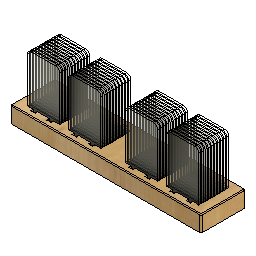
LED-Nixie-Clock (Autodesk Fusion 360 design; units mm, degrees)
Autodesk Fusion 360 part; units mm, degrees
note: some values were not read from the file. Chosen so that the rebuilt part matches the saved one: which face or edge a step refers to; how an offset face is resized. Set by a fixed rule: which sketch regions a step uses.
sketch "Skizze1" plane through (0, 0, 0) normal (0, 0, 1) x (1, 0, 0) in component "Digit"
  line L0 (-15, 60) -> (15, 60)
  line L1 (20, 55) -> (20, 0)
  line L2 (-20, 55) -> (-20, 0)
  line L3 (-20, 0) -> (-20, -10)
  line L4 (-20, -10) -> (20, -10)
  line L5 (20, -10) -> (20, 0)
  line L6 (-20, 0) -> (20, 0)
  arc A0 (-15, 60) -> (-20, 55) centre (-15, 55) ccw
  arc A1 (20, 55) -> (15, 60) centre (15, 55) ccw
  circle A2 centre (-10, -4.35) radius 1.65
  circle A3 centre (10, -4.35) radius 1.65
  line L7 (-20, -6) -> (20, -6) construction
  dimension "d8" = 10
  dimension "d9" = 5
  dimension "d10" = 5
  dimension "d11" = 60
  dimension "d12" = 40
  dimension "d96" = 3.3
  dimension "d97" = 3.3
  dimension "d124" = 6
  measures "d8" distance of origin
  measures "d9" radius of A0
  measures "d10" radius of A1
  measures "d11" distance of L0 L6
  measures "d12" distance of L1 L2
  measures "d96" diameter of A2
  measures "d97" diameter of A3
  measures "d124" distance of L6 L7
extrude "Extrusion1" add sketch "Skizze1" along normal blind 2.5 makes body 1 in component "Digit"
sketch "Skizze1 (2)" plane through (0, 0, 2.5) normal (0, 0, 1) x (-1, 0, 0) in component "Digit Spacer"
  circle A0 centre (10, 4.35) radius 1.65
  circle A1 centre (-10, 4.35) radius 1.65
  arc A2 (15, -60) -> (20, -55) centre (15, -55) ccw
  line L0 (20, -55) -> (20, 0)
  line L1 (20, 0) -> (20, 10)
  line L2 (20, 10) -> (-20, 10)
  line L3 (-20, 10) -> (-20, -55)
  arc A3 (-20, -55) -> (-15, -60) centre (-15, -55) ccw
  line L4 (-15, -60) -> (15, -60)
  circle A4 centre (10, 4.35) radius 1.65
  circle A5 centre (-10, 4.35) radius 1.65
  line L5 (20, 0) -> (-20, 0)
  line L6 (-20, 10) -> (-20, 0)
  line L7 (20, 10) -> (-20, 10)
  line L8 (20, 0) -> (20, 10)
extrude "Extrusion1'" add sketch "Skizze1 (2)" along normal blind 1.31 separate body contours L1 L2 L3 L5 L6 L7 L8 makes body 2 in component "Digit Spacer"
pattern_linear "R-Anordnung3" [suppressed]
pattern_linear "R-Anordnung6" [suppressed]
sketch "Skizze1 (3)" plane through (0, 0, 0) normal (0, 0, 1) x (1, 0, 0) in component "Digit Screw"
  circle A0 centre (0, 0) radius 1.5
  circle A1 centre (0, 0) radius 2.75
  line L0 (1.4382, 0.1218) -> (0.6136, 1.3064)
  line L1 (0.6136, 1.3064) -> (-0.8246, 1.1846)
  line L2 (-0.8246, 1.1846) -> (-1.4382, -0.1218)
  line L3 (-1.4382, -0.1218) -> (-0.6136, -1.3064)
  line L4 (-0.6136, -1.3064) -> (0.8246, -1.1846)
  line L5 (0.8246, -1.1846) -> (1.4382, 0.1218)
  line L6 (1.4064, 2.847) -> (-1.7623, 2.6415)
  line L7 (-1.7623, 2.6415) -> (-3.1688, -0.2055)
  line L8 (-3.1688, -0.2055) -> (-1.4064, -2.847)
  line L9 (-1.4064, -2.847) -> (1.7623, -2.6415)
  line L10 (1.7623, -2.6415) -> (3.1688, 0.2055)
  line L11 (3.1688, 0.2055) -> (1.4064, 2.847)
  dimension "d107" = 3
  dimension "d108" = 5.5
  dimension "d109" = 1.25
  dimension "d116" = 2.75
  measures "d107" diameter of A0
  measures "d108" diameter of A1
  measures "d109" distance of A0.centre L5
  measures "d116" distance of A0.centre L11
extrude "Extrusion1''" add sketch "Skizze1 (3)" against normal blind 3 separate body contours A0 | A1 makes body 3 in component "Digit Screw"
extrude "Extrusion2" add sketch "Skizze1 (3)" along normal blind 40 contours A0 | L0 L1 L2 L3 L4 L5 bodies 3 in component "Digit Screw"
thread "Gewinde1" "ISO Metric profile 3.0 M3x0.5 6g" major diameter 2.927 minor diameter 2.3555 pitch 0.5 angle 60 resizes the face on face at (1.4981, -0.0748, 26.6667) on bodies 3 in component "Digit Screw"
extrude "Extrusion3" add sketch "Skizze1 (3)" along normal blind 2.4 from surface at 36.79 separate body contours A1 | A1 L10 L11 | A1 L6 L11 | A1 L9 L10 | A1 L6 L7 | A1 L8 L9 | A1 L7 L8 makes body 4 in component "Digit Screw"
pattern_linear "R-Anordnung4" [suppressed]
pattern_linear "R-Anordnung5" [suppressed]
sketch "Skizze1 (4)" plane through (0, 0, 0) normal (0, 0, 1) x (1, 0, 0) in component "Base"
  line L0 (-20, 0) -> (-20, -36.79)
  line L1 (191.45, -36.79) -> (191.45, 0)
  line L2 (-31.775, 9.105) -> (203.225, 9.105)
  line L3 (203.225, 9.105) -> (203.225, -45.895)
  line L4 (203.225, -45.895) -> (-31.775, -45.895)
  line L5 (-31.775, -45.895) -> (-31.775, 9.105)
  line L6 (-12.75, -39.79) -> (-7.25, -39.79)
  line L7 (7.25, -39.79) -> (12.75, -39.79)
  line L8 (38.05, -39.79) -> (43.55, -39.79)
  line L9 (58.05, -39.79) -> (63.55, -39.79)
  line L10 (107.9, -39.79) -> (113.4, -39.79)
  line L11 (127.9, -39.79) -> (133.4, -39.79)
  line L12 (158.7, -39.79) -> (164.2, -39.79)
  line L13 (178.7, -39.79) -> (184.2, -39.79)
  line L14 (-12.75, -39.79) -> (-12.75, -36.79)
  line L15 (-7.25, -39.79) -> (-7.25, -36.79)
  line L16 (7.25, -39.79) -> (7.25, -36.79)
  line L17 (12.75, -36.79) -> (12.75, -39.79)
  line L18 (38.05, -36.79) -> (38.05, -39.79)
  line L19 (43.55, -39.79) -> (43.55, -36.79)
  line L20 (58.05, -39.79) -> (58.05, -36.79)
  line L21 (63.55, -36.79) -> (63.55, -39.79)
  line L22 (107.9, -36.79) -> (107.9, -39.79)
  line L23 (113.4, -39.79) -> (113.4, -36.79)
  line L24 (127.9, -36.79) -> (127.9, -39.79)
  line L25 (133.4, -39.79) -> (133.4, -36.79)
  line L26 (158.7, -36.79) -> (158.7, -39.79)
  line L27 (164.2, -36.79) -> (164.2, -39.79)
  line L28 (178.7, -36.79) -> (178.7, -39.79)
  line L29 (184.2, -39.79) -> (184.2, -36.79)
  line L30 (20, 0) -> (20, -36.79)
  line L31 (-20, 0) -> (20, 0)
  line L32 (30.8, 0) -> (30.8, -36.79)
  line L33 (70.8, -36.79) -> (70.8, 0)
  line L34 (70.8, 0) -> (30.8, 0)
  line L35 (100.65, -36.79) -> (100.65, 0)
  line L36 (100.65, 0) -> (140.65, 0)
  line L37 (140.65, 0) -> (140.65, -36.79)
  line L38 (151.45, -36.79) -> (151.45, 0)
  line L39 (151.45, 0) -> (191.45, 0)
  line L40 (-21.775, 3.605) -> (193.225, 3.605)
  line L41 (193.225, 3.605) -> (193.225, -40.395)
  line L42 (193.225, -40.395) -> (-21.775, -40.395)
  line L43 (-21.775, -40.395) -> (-21.775, 3.605)
  line L44 (85.725, 0) -> (85.725, 3.605) construction
  line L45 (70.8, 0) -> (100.65, 0) construction
  line L46 (85.725, 3.605) -> (85.725, 9.105) construction
  line L47 (-20, -18.395) -> (-21.775, -18.395) construction
  line L48 (-21.775, -18.395) -> (-31.775, -18.395) construction
  line L49 (-20, -18.395) -> (20, -18.395) construction
  line L50 (-12.75, 3) -> (-12.75, 0)
  line L51 (-12.75, 3) -> (-7.25, 3)
  line L52 (-7.25, 3) -> (-7.25, 0)
  line L53 (7.25, 3) -> (7.25, 0)
  line L54 (7.25, 3) -> (12.75, 3)
  line L55 (12.75, 0) -> (12.75, 3)
  line L56 (30.8, -18.395) -> (70.8, -18.395) construction
  line L57 (100.65, -18.395) -> (140.65, -18.395) construction
  line L58 (151.45, -18.395) -> (191.45, -18.395) construction
  line L59 (38.05, 0) -> (38.05, 3)
  line L60 (38.05, 3) -> (43.55, 3)
  line L61 (43.55, 3) -> (43.55, 0)
  line L62 (58.05, 3) -> (58.05, 0)
  line L63 (58.05, 3) -> (63.55, 3)
  line L64 (63.55, 0) -> (63.55, 3)
  line L65 (107.9, 0) -> (107.9, 3)
  line L66 (107.9, 3) -> (113.4, 3)
  line L67 (113.4, 3) -> (113.4, 0)
  line L68 (127.9, 0) -> (127.9, 3)
  line L69 (127.9, 3) -> (133.4, 3)
  line L70 (133.4, 3) -> (133.4, 0)
  line L71 (158.7, 0) -> (158.7, 3)
  line L72 (158.7, 3) -> (164.2, 3)
  line L73 (164.2, 0) -> (164.2, 3)
  line L74 (178.7, 0) -> (178.7, 3)
  line L75 (178.7, 3) -> (184.2, 3)
  line L76 (184.2, 3) -> (184.2, 0)
  line L77 (-20, -36.79) -> (20, -36.79)
  line L78 (30.8, -36.79) -> (70.8, -36.79)
  line L79 (100.65, -36.79) -> (140.65, -36.79)
  line L80 (151.45, -36.79) -> (191.45, -36.79)
  dimension "d122" = 55
  dimension "d123" = 235
  dimension "d147" = 215
  dimension "d148" = 44
  measures "d122" distance of origin
  measures "d148" distance of origin
extrude "Extrusion6" add sketch "Skizze1 (4)" against normal blind 20 separate body contours L0 L30 L31 L77 | L31 L50 L51 L52 | L6 L14 L15 L77 | L31 L53 L54 L55 | L7 L16 L17 L77 | L1 L38 L39 L80 | L13 L28 L29 L80 | L39 L74 L75 L76 | L12 L26 L27 L80 | L39 L71 L72 L73 | L2 L3 L4 L5 | L8 L18 L19 L78 | L32 L33 L34 L78 | L9 L20 L21 L78 | L34 L59 L60 L61 | L34 L62 L63 L64 | L10 L22 L23 L79 | L35 L36 L37 L79 | L11 L24 L25 L79 | L36 L65 L66 L67 | L36 L68 L69 L70 | L40 L41 L42 L43 makes body 5 in component "Base"
extrude "Extrusion9" cut sketch "Skizze1 (4)" against normal blind 10 contours L0 L30 L31 L77 | L1 L38 L39 L80 | L32 L33 L34 L78 | L35 L36 L37 L79 bodies 5 in component "Base"
extrude "Extrusion10" cut sketch "Skizze1 (4)" against normal blind 7.5 contours L31 L50 L51 L52 | L6 L14 L15 L77 | L31 L53 L54 L55 | L7 L16 L17 L77 | L13 L28 L29 L80 | L39 L74 L75 L76 | L12 L26 L27 L80 | L39 L71 L72 L73 | L8 L18 L19 L78 | L9 L20 L21 L78 | L34 L59 L60 L61 | L34 L62 L63 L64 | L10 L22 L23 L79 | L11 L24 L25 L79 | L36 L65 L66 L67 | L36 L68 L69 L70 bodies 5 in component "Base"
extrude "Extrusion11" cut sketch "Skizze1 (4)" against normal blind 10 from surface at -10 contours L0 L30 L31 L77 | L31 L50 L51 L52 | L6 L14 L15 L77 | L31 L53 L54 L55 | L7 L16 L17 L77 | L1 L38 L39 L80 | L13 L28 L29 L80 | L39 L74 L75 L76 | L12 L26 L27 L80 | L39 L71 L72 L73 | L8 L18 L19 L78 | L32 L33 L34 L78 | L9 L20 L21 L78 | L34 L59 L60 L61 | L34 L62 L63 L64 | L10 L22 L23 L79 | L35 L36 L37 L79 | L11 L24 L25 L79 | L36 L65 L66 L67 | L36 L68 L69 L70 | L40 L41 L42 L43 bodies 5 in component "Base"
hole "Bohrung2" at (76.3217, 9.105, -19.9759) direction (0, -1, 0) diameter 10 depth 10 tip angle 180 bodies 5 in component "Base"
fillet "Abrundung2" radius 2 4 edges at (-31.775, -45.895, -10) (-31.775, 9.105, -10) (203.225, 9.105, -10) (203.225, -45.895, -10) on bodies 5 in component "Base"
chamfer "Fase2" distance 1 angle 45 8 edges at (-31.775, -18.395, 0) (-31.1892, 8.5192, 0) (85.725, 9.105, 0) (202.6392, 8.5192, 0) (203.225, -18.395, 0) (202.6392, -45.3092, 0) (85.725, -45.895, 0) (-31.1892, -45.3092, 0) on bodies 5 in component "Base"
sketch "Skizze1 (5)" plane through (0, 0, 0) normal (0, 0, 1) x (1, 0, 0) in component "PCB"
  line L0 (0, 0) -> (214.63, 0)
  line L1 (214.63, 0) -> (214.63, -43.18)
  line L2 (214.63, -43.18) -> (0, -43.18)
  line L3 (0, -43.18) -> (0, 0)
  line L4 (107.315, 0) -> (107.315, -43.18) construction
  line L5 (0, -3.17) -> (214.63, -3.17) construction
  line L6 (0, -40.01) -> (214.63, -40.01) construction
  circle A0 centre (107.315, -3.17) radius 1.65
  circle A1 centre (107.315, -40.01) radius 1.65
  line L7 (46.985, 0) -> (46.985, -43.18) construction
  line L8 (167.645, 0) -> (167.645, -43.18) construction
  circle A2 centre (46.985, -3.17) radius 1.65
  circle A3 centre (46.985, -40.01) radius 1.65
  circle A4 centre (167.645, -3.17) radius 1.65
  circle A5 centre (167.645, -40.01) radius 1.65
  dimension "d154" = 43.18
  dimension "d155" = 214.63
  dimension "d156" = 3.17
  dimension "d157" = 3.17
  dimension "d158" = 3.3
  dimension "d159" = 3.3
  dimension "d160" = 60.33
  dimension "d161" = 60.33
  dimension "d162" = 3.3
  dimension "d163" = 3.3
  dimension "d164" = 3.3
  dimension "d165" = 3.3
  measures "d154" distance of L0.start
  measures "d155" distance of L0.start
  measures "d156" distance of L0 L5
  measures "d157" distance of L2 L6
  measures "d158" diameter of A0
  measures "d159" diameter of A1
  measures "d160" distance of L4 L7
  measures "d161" distance of L4 L8
  measures "d162" diameter of A2
  measures "d163" diameter of A3
  measures "d164" diameter of A4
  measures "d165" diameter of A5
extrude "Extrusion1'''" add sketch "Skizze1 (5)" along normal blind 1.6 separate body makes body 6 in component "PCB"
component "Digit" placed x (1, 0, 0) y (0, 0, 1) z (0, -1, 0) at (0, 0, 0)
component "Digit Spacer" placed x (1, 0, 0) y (0, 0, 1) z (0, -1, 0) at (0, 0, 0)
component "Digit" placed x (1, 0, 0) y (0, 0, 1) z (0, -1, 0) at (0, -3.81, 0)
component "Digit" placed x (1, 0, 0) y (0, 0, 1) z (0, -1, 0) at (0, -7.62, 0)
component "Digit" placed x (1, 0, 0) y (0, 0, 1) z (0, -1, 0) at (0, -11.43, 0)
component "Digit" placed x (1, 0, 0) y (0, 0, 1) z (0, -1, 0) at (0, -15.24, 0)
component "Digit" placed x (1, 0, 0) y (0, 0, 1) z (0, -1, 0) at (0, -19.05, 0)
component "Digit" placed x (1, 0, 0) y (0, 0, 1) z (0, -1, 0) at (0, -22.86, 0)
component "Digit" placed x (1, 0, 0) y (0, 0, 1) z (0, -1, 0) at (0, -26.67, 0)
component "Digit" placed x (1, 0, 0) y (0, 0, 1) z (0, -1, 0) at (0, -30.48, 0)
component "Digit" placed x (1, 0, 0) y (0, 0, 1) z (0, -1, 0) at (0, -34.29, 0)
component "Digit Spacer" placed x (1, 0, 0) y (0, 0, 1) z (0, -1, 0) at (0, -3.81, 0)
component "Digit Spacer" placed x (1, 0, 0) y (0, 0, 1) z (0, -1, 0) at (0, -7.62, 0)
component "Digit Spacer" placed x (1, 0, 0) y (0, 0, 1) z (0, -1, 0) at (0, -11.43, 0)
component "Digit Spacer" placed x (1, 0, 0) y (0, 0, 1) z (0, -1, 0) at (0, -15.24, 0)
component "Digit Spacer" placed x (1, 0, 0) y (0, 0, 1) z (0, -1, 0) at (0, -19.05, 0)
component "Digit Spacer" placed x (1, 0, 0) y (0, 0, 1) z (0, -1, 0) at (0, -22.86, 0)
component "Digit Spacer" placed x (1, 0, 0) y (0, 0, 1) z (0, -1, 0) at (0, -26.67, 0)
component "Digit Spacer" placed x (1, 0, 0) y (0, 0, 1) z (0, -1, 0) at (0, -30.48, 0)
component "Digit Screw" placed x (1, 0, 0) y (0, 0, -1) z (0, 1, 0) at (-10, -36.79, -5)
component "Digit Screw" placed x (1, 0, 0) y (0, 0, -1) z (0, 1, 0) at (10, -36.79, -5)
component "Digit" placed x (1, 0, 0) y (0, 0, 1) z (0, -1, 0) at (50.8, 0, 0)
component "Digit Spacer" placed x (1, 0, 0) y (0, 0, 1) z (0, -1, 0) at (50.8, 0, 0)
component "Digit" placed x (1, 0, 0) y (0, 0, 1) z (0, -1, 0) at (50.8, -3.81, 0)
component "Digit" placed x (1, 0, 0) y (0, 0, 1) z (0, -1, 0) at (50.8, -7.62, 0)
component "Digit" placed x (1, 0, 0) y (0, 0, 1) z (0, -1, 0) at (50.8, -11.43, 0)
component "Digit" placed x (1, 0, 0) y (0, 0, 1) z (0, -1, 0) at (50.8, -15.24, 0)
component "Digit" placed x (1, 0, 0) y (0, 0, 1) z (0, -1, 0) at (50.8, -19.05, 0)
component "Digit" placed x (1, 0, 0) y (0, 0, 1) z (0, -1, 0) at (50.8, -22.86, 0)
component "Digit" placed x (1, 0, 0) y (0, 0, 1) z (0, -1, 0) at (50.8, -26.67, 0)
component "Digit" placed x (1, 0, 0) y (0, 0, 1) z (0, -1, 0) at (50.8, -30.48, 0)
component "Digit" placed x (1, 0, 0) y (0, 0, 1) z (0, -1, 0) at (50.8, -34.29, 0)
component "Digit Spacer" placed x (1, 0, 0) y (0, 0, 1) z (0, -1, 0) at (50.8, -3.81, 0)
component "Digit Spacer" placed x (1, 0, 0) y (0, 0, 1) z (0, -1, 0) at (50.8, -7.62, 0)
component "Digit Spacer" placed x (1, 0, 0) y (0, 0, 1) z (0, -1, 0) at (50.8, -11.43, 0)
component "Digit Spacer" placed x (1, 0, 0) y (0, 0, 1) z (0, -1, 0) at (50.8, -15.24, 0)
component "Digit Spacer" placed x (1, 0, 0) y (0, 0, 1) z (0, -1, 0) at (50.8, -19.05, 0)
component "Digit Spacer" placed x (1, 0, 0) y (0, 0, 1) z (0, -1, 0) at (50.8, -22.86, 0)
component "Digit Spacer" placed x (1, 0, 0) y (0, 0, 1) z (0, -1, 0) at (50.8, -26.67, 0)
component "Digit Spacer" placed x (1, 0, 0) y (0, 0, 1) z (0, -1, 0) at (50.8, -30.48, 0)
component "Digit Screw" placed x (1, 0, 0) y (0, 0, -1) z (0, 1, 0) at (40.8, -36.79, -5)
component "Digit Screw" placed x (1, 0, 0) y (0, 0, -1) z (0, 1, 0) at (60.8, -36.79, -5)
component "Digit" placed x (1, 0, 0) y (0, 0, 1) z (0, -1, 0) at (120.65, 0, 0)
component "Digit" placed x (1, 0, 0) y (0, 0, 1) z (0, -1, 0) at (171.45, 0, 0)
component "Digit Spacer" placed x (1, 0, 0) y (0, 0, 1) z (0, -1, 0) at (120.65, 0, 0)
component "Digit" placed x (1, 0, 0) y (0, 0, 1) z (0, -1, 0) at (120.65, -3.81, 0)
component "Digit" placed x (1, 0, 0) y (0, 0, 1) z (0, -1, 0) at (120.65, -7.62, 0)
component "Digit" placed x (1, 0, 0) y (0, 0, 1) z (0, -1, 0) at (120.65, -11.43, 0)
component "Digit" placed x (1, 0, 0) y (0, 0, 1) z (0, -1, 0) at (120.65, -15.24, 0)
component "Digit" placed x (1, 0, 0) y (0, 0, 1) z (0, -1, 0) at (120.65, -19.05, 0)
component "Digit" placed x (1, 0, 0) y (0, 0, 1) z (0, -1, 0) at (120.65, -22.86, 0)
component "Digit" placed x (1, 0, 0) y (0, 0, 1) z (0, -1, 0) at (120.65, -26.67, 0)
component "Digit" placed x (1, 0, 0) y (0, 0, 1) z (0, -1, 0) at (120.65, -30.48, 0)
component "Digit" placed x (1, 0, 0) y (0, 0, 1) z (0, -1, 0) at (120.65, -34.29, 0)
component "Digit Spacer" placed x (1, 0, 0) y (0, 0, 1) z (0, -1, 0) at (120.65, -3.81, 0)
component "Digit Spacer" placed x (1, 0, 0) y (0, 0, 1) z (0, -1, 0) at (120.65, -7.62, 0)
component "Digit Spacer" placed x (1, 0, 0) y (0, 0, 1) z (0, -1, 0) at (120.65, -11.43, 0)
component "Digit Spacer" placed x (1, 0, 0) y (0, 0, 1) z (0, -1, 0) at (120.65, -15.24, 0)
component "Digit Spacer" placed x (1, 0, 0) y (0, 0, 1) z (0, -1, 0) at (120.65, -19.05, 0)
component "Digit Spacer" placed x (1, 0, 0) y (0, 0, 1) z (0, -1, 0) at (120.65, -22.86, 0)
component "Digit Spacer" placed x (1, 0, 0) y (0, 0, 1) z (0, -1, 0) at (120.65, -26.67, 0)
component "Digit Spacer" placed x (1, 0, 0) y (0, 0, 1) z (0, -1, 0) at (120.65, -30.48, 0)
component "Digit Screw" placed x (1, 0, 0) y (0, 0, -1) z (0, 1, 0) at (110.65, -36.79, -5)
component "Digit Screw" placed x (1, 0, 0) y (0, 0, -1) z (0, 1, 0) at (130.65, -36.79, -5)
component "Digit Spacer" placed x (1, 0, 0) y (0, 0, 1) z (0, -1, 0) at (171.45, 0, 0)
component "Digit" placed x (1, 0, 0) y (0, 0, 1) z (0, -1, 0) at (171.45, -3.81, 0)
component "Digit" placed x (1, 0, 0) y (0, 0, 1) z (0, -1, 0) at (171.45, -7.62, 0)
component "Digit" placed x (1, 0, 0) y (0, 0, 1) z (0, -1, 0) at (171.45, -11.43, 0)
component "Digit" placed x (1, 0, 0) y (0, 0, 1) z (0, -1, 0) at (171.45, -15.24, 0)
component "Digit" placed x (1, 0, 0) y (0, 0, 1) z (0, -1, 0) at (171.45, -19.05, 0)
component "Digit" placed x (1, 0, 0) y (0, 0, 1) z (0, -1, 0) at (171.45, -22.86, 0)
component "Digit" placed x (1, 0, 0) y (0, 0, 1) z (0, -1, 0) at (171.45, -26.67, 0)
component "Digit" placed x (1, 0, 0) y (0, 0, 1) z (0, -1, 0) at (171.45, -30.48, 0)
component "Digit" placed x (1, 0, 0) y (0, 0, 1) z (0, -1, 0) at (171.45, -34.29, 0)
component "Digit Spacer" placed x (1, 0, 0) y (0, 0, 1) z (0, -1, 0) at (171.45, -3.81, 0)
component "Digit Spacer" placed x (1, 0, 0) y (0, 0, 1) z (0, -1, 0) at (171.45, -7.62, 0)
component "Digit Spacer" placed x (1, 0, 0) y (0, 0, 1) z (0, -1, 0) at (171.45, -11.43, 0)
component "Digit Spacer" placed x (1, 0, 0) y (0, 0, 1) z (0, -1, 0) at (171.45, -15.24, 0)
component "Digit Spacer" placed x (1, 0, 0) y (0, 0, 1) z (0, -1, 0) at (171.45, -19.05, 0)
component "Digit Spacer" placed x (1, 0, 0) y (0, 0, 1) z (0, -1, 0) at (171.45, -22.86, 0)
component "Digit Spacer" placed x (1, 0, 0) y (0, 0, 1) z (0, -1, 0) at (171.45, -26.67, 0)
component "Digit Spacer" placed x (1, 0, 0) y (0, 0, 1) z (0, -1, 0) at (171.45, -30.48, 0)
component "Digit Screw" placed x (1, 0, 0) y (0, 0, -1) z (0, 1, 0) at (161.45, -36.79, -5)
component "Digit Screw" placed x (1, 0, 0) y (0, 0, -1) z (0, 1, 0) at (181.45, -36.79, -5)
component "Base" placed x (1, 0, 0) y (0, 1, 0) z (0, 0, 1) at (0, 0, 0)
component "PCB" placed x (1, 0, 0) y (0, 1, 0) z (0, 0, 1) at (-21.5614, 3.2122, -11.6)
equation "digit_width = 40 mm" comment "Width of acrylic digits"
equation "digit_height = 60 mm" comment "Height of acrylic digits"
equation "digit_thickness = 2.5 mm" comment "Thickness of acrylic digits"
equation "d9 = digit_roundness"
equation "d10 = digit_roundness"
equation "d11 = digit_height"
equation "d12 = digit_width"
equation "digit_roundness = 5 mm" comment "Roundness of acrylic digits (radius)"
equation "d14 = digit_thickness"
equation "led_width = 5 mm" comment "Width and height of LEDs"
equation "digit_spacing = 1.31 mm" comment "Spacing of acrylic digit plates (depth)"
equation "digit_distance = 10.8 mm" comment "Distance between an acrylic digit and its left/right neighbours"
equation "extra_spacing = 0.1 mm" comment "Extra spacing for fitting components into others"
equation "d85 = digit_thickness + digit_spacing"
equation "d89 = digit_width + digit_distance"
equation "d93 = 2 * digit_width + digit_distance + mid_distance"
equation "d101 = digit_spacing"
equation "d105 = digit_thickness + digit_spacing"
equation "d117 = 10 * digit_thickness + 9 * digit_spacing"
equation "mid_distance = 29.85 mm" comment "Distance between hour digits and minute digits"
